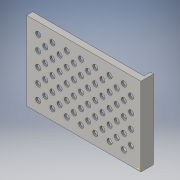
# Autodesk Inventor part: RaspPiCaseTop
Saved by Autodesk Inventor 2016 (Build 200138000, 138)
## iProperties
Created: 2016-04-29
Part Number: RaspPiCaseTop
Material: Generic
Document SubType Name: Modeling
Designer: mkepler
Density: 1 g/cm^3
Appearance: Default
Author: mkepler
Autodesk Inventor part; units mm, degrees
ref_plane "YZ Plane" through (0, 0, 0) normal (1, 0, 0) x (0, 1, 0)
ref_plane "XZ Plane" through (0, 0, 0) normal (0, 1, 0) x (-1, 0, 0)
ref_plane "XY Plane" through (0, 0, 0) normal (0, 0, 1) x (1, 0, 0)
sketch "Sketch1" plane through (0, 0, 0) normal (0, 1, 0) x (-1, 0, 0)
  line L0 (0, 0) -> (91.5, 0)
  line L1 (91.5, 0) -> (91.5, -63)
  line L2 (91.5, -63) -> (0, -63)
  circle A0 centre (84, -7.5) radius 2.15
  circle A1 centre (84, -19.5) radius 2.15
  circle A2 centre (84, -31.5) radius 2.15
  circle A3 centre (84, -55.5) radius 2.15
  circle A4 centre (84, -43.5) radius 2.15
  circle A5 centre (78, -13.5) radius 2.15
  circle A6 centre (78, -25.5) radius 2.15
  circle A7 centre (78, -37.5) radius 2.15
  circle A8 centre (78, -49.5) radius 2.15
  circle A9 centre (66, -13.5) radius 2.15
  circle A10 centre (66, -25.5) radius 2.15
  circle A11 centre (66, -37.5) radius 2.15
  circle A12 centre (66, -49.5) radius 2.15
  circle A13 centre (72, -31.5) radius 2.15
  circle A14 centre (72, -19.5) radius 2.15
  circle A15 centre (72, -7.5) radius 2.15
  circle A16 centre (72, -55.5) radius 2.15
  circle A17 centre (72, -43.5) radius 2.15
  line L3 (66, -55.5) -> (63, -55.5)
  line L4 (63, -55.5) -> (63, -45.305)
  circle A18 centre (42, -13.5) radius 2.15
  circle A19 centre (42, -25.5) radius 2.15
  circle A20 centre (42, -37.5) radius 2.15
  circle A21 centre (42, -49.5) radius 2.15
  circle A22 centre (48, -31.5) radius 2.15
  circle A23 centre (48, -19.5) radius 2.15
  circle A24 centre (48, -7.5) radius 2.15
  circle A25 centre (48, -55.5) radius 2.15
  circle A26 centre (48, -43.5) radius 2.15
  circle A27 centre (54, -37.5) radius 2.15
  circle A28 centre (60, -31.5) radius 2.15
  circle A29 centre (54, -25.5) radius 2.15
  circle A30 centre (60, -19.5) radius 2.15
  circle A31 centre (54, -13.5) radius 2.15
  circle A32 centre (60, -7.5) radius 2.15
  circle A33 centre (60, -43.5) radius 2.15
  circle A34 centre (54, -49.5) radius 2.15
  circle A35 centre (60, -55.5) radius 2.15
  line L5 (42, -55.5) -> (39, -55.5)
  line L6 (39, -55.5) -> (39, -51.65)
  circle A36 centre (6, -37.5) radius 2.15
  circle A37 centre (12, -31.5) radius 2.15
  circle A38 centre (6, -25.5) radius 2.15
  circle A39 centre (12, -19.5) radius 2.15
  circle A40 centre (6, -13.5) radius 2.15
  circle A41 centre (12, -7.5) radius 2.15
  circle A42 centre (12, -43.5) radius 2.15
  circle A43 centre (6, -49.5) radius 2.15
  circle A44 centre (12, -55.5) radius 2.15
  line L7 (12, -55.5) -> (15, -55.5)
  line L8 (15, -55.5) -> (15, -45.305)
  circle A45 centre (36, -43.5) radius 2.15
  circle A46 centre (30, -49.5) radius 2.15
  circle A47 centre (24, -55.5) radius 2.15
  circle A48 centre (24, -43.5) radius 2.15
  circle A49 centre (36, -55.5) radius 2.15
  circle A50 centre (36, -7.5) radius 2.15
  circle A51 centre (30, -25.5) radius 2.15
  circle A52 centre (30, -13.5) radius 2.15
  circle A53 centre (18, -25.5) radius 2.15
  circle A54 centre (24, -19.5) radius 2.15
  circle A55 centre (18, -13.5) radius 2.15
  circle A56 centre (24, -7.5) radius 2.15
  circle A57 centre (36, -19.5) radius 2.15
  circle A58 centre (36, -31.5) radius 2.15
  circle A59 centre (30, -37.5) radius 2.15
  circle A60 centre (24, -31.5) radius 2.15
  circle A61 centre (18, -49.5) radius 2.15
  circle A62 centre (18, -37.5) radius 2.15
  line L9 (36, -55.5) -> (39, -55.5)
  line L10 (0, 0) -> (0, -63)
  dimension "d0" = 91.5
  dimension "d1" = 63
  dimension "d2" = 4.3
  dimension "d3" = 7.5
  dimension "d4" = 7.5
  dimension "d11" = 4.3
  dimension "d17" = 3
  dimension "d18" = 3
  constraints: 63 centre point, 22 end point, 6 symmetric about line, 3 horizontal, 3 perpendicular, 1 parallel, 1 vertical
  measures "d0" distance of L1.end L2.end
  measures "d1" distance of L0.end L1.end
  measures "d2" diameter of A0
  measures "d3" distance from line of L0 A0.centre
  measures "d4" distance from line of L1 A0.centre
  measures "d11" diameter of A2
  measures "d17" distance of L3.start L3.end
  measures "d18" distance of L5.start L5.end
extrude "Extrusion1" add sketch "Sketch1" along normal blind 1.5
sketch "Sketch2" plane through (0, 1.5, 0) normal (0, 1, 0) x (1, 0, 0)
  line L0 (3, 0) -> (3, -3)
  line L1 (3, -3) -> (-94.5, -3)
  line L2 (-94.5, -3) -> (-94.5, 66)
  line L3 (-94.5, 66) -> (3, 66)
  line L4 (3, 66) -> (3, 0)
  line L5 (-91.5, 63) -> (-91.5, 0) projected
  line L6 (0, 63) -> (-91.5, 63) projected
  line L7 (-91.5, 0) -> (0, 0)
  line L8 (0, 0) -> (0, 63)
  line L9 (0, 63) -> (-91.5, 63)
  line L10 (-91.5, 63) -> (-91.5, 0)
  dimension "d30" = 97.5
  dimension "d31" = 69
  dimension "d32" = 97.5
  constraints: 18 end point, 3 perpendicular, 2 parallel, 1 horizontal, 1 vertical
  measures "d30" distance of L0.end L1.end
  measures "d31" distance of L1.end L2.end
  measures "d32" distance of L2.end L3.end
extrude "Extrusion2" add sketch "Sketch2" along normal blind 3.612 and the other way blind 1.5
sketch "Sketch5" plane through (0, 1.5, 0) normal (0, 1, 0) x (1, 0, 0)
  point P0 (0, 0)
sketch "Sketch6" plane through (0, 5.112, 0) normal (0, 1, 0) x (1, 0, 0)
  line L0 (0, 0) -> (0, 63) projected
  line L1 (3, 66) -> (3, -3) projected
  line L2 (0, 0) -> (3, 0)
  line L3 (3, 0) -> (3, 63)
  line L4 (3, 63) -> (0, 63)
  line L5 (0, 63) -> (0, 0)
  constraints: 8 end point, 2 parallel, 1 horizontal, 1 perpendicular, 1 point on line
extrude "Extrusion3" add sketch "Sketch6" along normal blind 5.388
sketch "Sketch7" plane through (-91.5, 1.5, -63) normal (0, 0, 1) x (1, 0, 0)
  point P0 (91.5, -1.5)
sketch "Sketch8" plane through (-91.5, 1.5, -63) normal (0, 0, 1) x (1, 0, 0)
  line L0 (91.5, 0) -> (0, 0) projected
  line L1 (0, 3.612) -> (91.5, 3.612) projected
  line L2 (0, 0) -> (91.5, 0)
  line L3 (91.5, 0) -> (91.5, 3.612)
  line L4 (91.5, 3.612) -> (0, 3.612)
  line L5 (0, 3.612) -> (0, 0)
  point P0 (91.5, -1.5)
  constraints: 8 end point, 2 parallel, 1 horizontal, 1 perpendicular
extrude "Extrusion4" cut sketch "Sketch8" against normal blind 0.5
sketch "Sketch9" plane through (0, 1.5, 0) normal (0, 0, -1) x (-1, 0, 0)
  line L0 (0, 3.612) -> (91.5, 3.612) projected
  line L1 (91.5, 0) -> (0, 0) projected
  line L2 (91.5, 3.612) -> (0, 3.612)
  line L3 (0, 3.612) -> (0, 0)
  line L4 (0, 0) -> (91.5, 0)
  line L5 (91.5, 0) -> (91.5, 3.612)
  point P0 (0, -1.5)
  constraints: 8 end point, 2 parallel, 1 horizontal, 1 perpendicular
extrude "Extrusion5" cut sketch "Sketch9" against normal blind 0.5
sketch "Sketch10" plane through (-91.5, 1.5, -63.5) normal (1, 0, 0) x (0, 0, -1)
  line L0 (0, 0) -> (0, 3.612) projected
  line L1 (0, 0) -> (-64, 0) projected
  line L2 (0, 3.612) -> (-64, 3.612)
  line L3 (-64, 3.612) -> (-64, 0)
  line L4 (-64, 0) -> (0, 0)
  line L5 (0, 0) -> (0, 3.612)
  point P0 (-63.5, -1.5)
  constraints: 8 end point, 2 parallel, 1 horizontal, 1 perpendicular
extrude "Extrusion6" cut sketch "Sketch10" against normal blind 0.5
sketch "Sketch11" plane through (3, 5.112, -63) normal (0, 0, -1) x (-1, 0, 0)
  line L0 (0, 5.388) -> (3, 5.388) projected
  line L1 (0, 0) -> (0, 5.388) projected
  line L2 (3, 5.388) -> (0, 5.388)
  line L3 (0, 5.388) -> (0, 0)
  line L4 (0, 0) -> (3, 0)
  line L5 (3, 0) -> (3, 5.388)
  point P0 (3, -5.112)
  constraints: 8 end point, 2 parallel, 1 horizontal, 1 perpendicular
extrude "Extrusion7" add sketch "Sketch11" along normal blind 3
sketch "Sketch12" plane through (0, 5.112, 0) normal (0, 0, 1) x (1, 0, 0)
  line L0 (0, 5.388) -> (3, 5.388) projected
  line L1 (-94.5, 0) -> (3, 0) projected
  line L2 (0, 5.388) -> (3, 5.388)
  line L3 (3, 5.388) -> (3, 0)
  line L4 (3, 0) -> (0, 0)
  line L5 (0, 0) -> (0, 5.388)
  point P0 (0, -5.112)
  constraints: 8 end point, 2 parallel, 1 horizontal, 1 perpendicular
extrude "Extrusion8" add sketch "Sketch12" along normal blind 3
sketch "Sketch13" plane through (0, 0, 0) normal (0, -1, 0) x (1, 0, 0)
  line L0 (-94.5, 3) -> (0, 3) projected
  line L1 (-94.5, 3) -> (-93.75, 3)
  line L2 (-93.75, 1.5) -> (2.25, 1.5)
  line L3 (2.25, 1.5) -> (2.25, -64.5)
  line L4 (2.25, -64.5) -> (-93.75, -64.5)
  line L5 (-93.75, -64.5) -> (-93.75, 1.5)
  line L6 (3, -66) -> (3, 3) projected
  line L7 (-94.5, 3) -> (3, 3)
  line L8 (3, 3) -> (3, -66)
  line L9 (3, -66) -> (-94.5, -66)
  line L10 (-94.5, -66) -> (-94.5, 3)
  point P0 (0, 0)
  dimension "d45" = 0.75
  dimension "d46" = 1.5
  dimension "d47" = 96
  dimension "d48" = 66
  constraints: 18 end point, 4 parallel, 2 horizontal, 2 perpendicular, 1 point on line
  measures "d45" distance of L0.start L1.end
  measures "d46" distance of L1.end L2.start
  measures "d47" distance of L3.end L4.end
  measures "d48" distance of L2.end L3.end
extrude "Extrusion9" cut sketch "Sketch13" against normal through all
sketch "Sketch14" plane through (-93.75, 0, -64.5) normal (-1, 0, 0) x (0, 0, 1)
  line L0 (0, 5.112) -> (66, 5.112) projected
  line L1 (0, 0) -> (0, 5.112) projected
  line L2 (66, 5.112) -> (0, 5.112)
  line L3 (0, 5.112) -> (0, 1.5)
  line L4 (0, 1.5) -> (66, 1.5)
  line L5 (66, 1.5) -> (66, 5.112)
  point P0 (64.5, 0)
  constraints: 8 end point, 2 parallel, 1 horizontal, 1 perpendicular, 1 point on line
extrude "Extrusion10" cut sketch "Sketch14" against normal through all
sketch "Sketch15" plane through (0, 10.5, 1.5) normal (0, 0, 1) x (1, 0, 0)
  line L0 (2.25, -5.388) -> (2.25, 0) projected
  line L1 (0, -5.388) -> (0, 0) projected
  line L2 (2.25, -5.388) -> (0, -5.388)
  line L3 (0, -5.388) -> (0, 0)
  line L4 (0, 0) -> (2.25, 0)
  line L5 (2.25, 0) -> (2.25, -5.388)
  point P0 (0, -10.5)
  constraints: 8 end point, 2 parallel, 1 horizontal, 1 perpendicular
extrude "Extrusion11" cut sketch "Sketch15" against normal through all
sketch "Sketch16" plane through (0, 1.5, 0) normal (0, 1, 0) x (1, 0, 0)
  line L0 (2.25, 64.5) -> (2.25, -1.5) projected
  line L1 (2.25, -1.5) -> (-0.75, -1.5)
  line L2 (-0.75, -1.5) -> (-0.75, 3.5)
  line L3 (-0.75, 3.5) -> (2.25, 3.5)
  line L4 (2.25, 3.5) -> (2.25, -1.5)
  line L5 (2.25, 64.5) -> (-0.75, 64.5)
  line L6 (-0.75, 64.5) -> (-0.75, 59.5)
  line L7 (-0.75, 59.5) -> (2.25, 59.5)
  line L8 (2.25, 59.5) -> (2.25, 64.5)
  line L9 (2.25, 3.5) -> (-0.75, 3.5)
  line L10 (-0.75, 3.5) -> (-0.75, 59.5)
  line L11 (-0.75, 59.5) -> (2.25, 59.5)
  line L12 (2.25, 59.5) -> (2.25, 3.5)
  point P0 (0, 0)
  dimension "d55" = 3
  dimension "d56" = 5
  dimension "d57" = 3
  dimension "d58" = 5
  constraints: 24 end point, 6 parallel, 3 horizontal, 3 perpendicular
  measures "d55" distance of L2.end L3.end
  measures "d56" distance of L1.end L2.end
  measures "d57" distance of L7.end L6.end
  measures "d58" distance of L6.end L5.end
extrude "Extrusion12" add sketch "Sketch16" along normal blind 9
sketch "Sketch17" plane through (0, 1.5, 0) normal (0, 1, 0) x (1, 0, 0)
  line L0 (-0.75, -1.5) -> (-93.75, -1.5) projected
  line L1 (-0.75, -1.5) -> (-0.75, 0)
  line L2 (-0.75, -1.5) -> (-0.75, 64.5) projected
  line L3 (-93.75, -1.5) -> (-93.75, 64.5) projected
  line L4 (-93.75, -1.5) -> (-93.75, 64.5)
  line L5 (-93.75, 64.5) -> (-0.75, 64.5) projected
  line L6 (-93.75, 64.5) -> (-0.75, 64.5)
  line L7 (-0.75, 64.5) -> (-0.75, 63)
  line L8 (-92.25, 63) -> (-0.75, 63)
  line L9 (-0.75, 0) -> (-92.25, 0)
  line L10 (-92.25, 0) -> (-92.25, 63)
  point P0 (0, 0)
  dimension "d61" = 1.5
  constraints: 14 end point, 3 perpendicular, 2 point on line, 1 collinear, 1 parallel
  measures "d61" distance of L2.end L7.end
extrude "Extrusion13" add sketch "Sketch17" along normal blind 3.65 contours L0 L3 L5 L2 L8 L10 L9 L1
sketch "Sketch18" plane through (-0.75, 1.5, 0) normal (0, 0, -1) x (-1, 0, 0)
  line L0 (91.5, 0) -> (91.5, 3.65) projected
  line L1 (0, 0) -> (0, 3.65) projected
  line L2 (91.5, 3.65) -> (0, 3.65)
  line L3 (0, 3.65) -> (0, 0)
  line L4 (0, 0) -> (91.5, 0)
  line L5 (91.5, 0) -> (91.5, 3.65)
  point P0 (-0.75, -1.5)
  constraints: 8 end point, 2 parallel, 1 horizontal, 1 perpendicular
extrude "Extrusion14" cut sketch "Sketch18" against normal blind 0.5
sketch "Sketch19" plane through (-92.25, 1.5, -63) normal (0, 0, 1) x (1, 0, 0)
  line L0 (91.5, 0) -> (0, 0) projected
  line L1 (0, 0) -> (0, 3.65) projected
  line L2 (91.5, 0) -> (0, 0)
  line L3 (0, 0) -> (0, 3.65)
  line L4 (0, 3.65) -> (91.5, 3.65)
  line L5 (91.5, 3.65) -> (91.5, 0)
  point P0 (92.25, -1.5)
  constraints: 8 end point, 2 parallel, 1 horizontal, 1 perpendicular
extrude "Extrusion15" cut sketch "Sketch19" against normal blind 0.5
sketch "Sketch20" plane through (-92.25, 1.5, 0.5) normal (1, 0, 0) x (0, 0, -1)
  line L0 (64, 0) -> (64, 3.65) projected
  line L1 (64, 0) -> (0, 0)
  line L2 (0, 0) -> (0, 3.65)
  line L3 (0, 3.65) -> (64, 3.65)
  line L4 (64, 3.65) -> (64, 0)
  point P0 (0.5, -1.5)
  constraints: 8 end point, 2 parallel, 1 horizontal, 1 perpendicular
extrude "Extrusion16" cut sketch "Sketch20" against normal blind 0.5
sketch "Sketch21" plane through (-0.75, 10.5, -64.5) normal (-1, 0, 0) x (0, 0, 1)
  line L0 (1, -5.35) -> (1, -9) projected
  line L1 (1, -9) -> (1, -5.35)
  line L2 (0, -5.35) -> (1, -5.35) projected
  line L3 (1, -5.35) -> (0, -5.35)
  line L4 (0, -5.35) -> (0, 0)
  line L5 (66, -5.35) -> (66, 0) projected
  line L6 (0, 0) -> (66, 0)
  line L7 (65, -5.35) -> (66, -5.35) projected
  line L8 (66, -5.4693) -> (65, -5.35)
  line L9 (65, -9) -> (65, -5.35) projected
  line L10 (65, -5.35) -> (65, -9)
  line L11 (65, -5.35) -> (66, -5.35)
  line L12 (66, -5.35) -> (66, 0)
  line L13 (65, -9) -> (1, -9) projected
  line L14 (65, -9) -> (1, -9)
  line L15 (1, -9) -> (1, -5.35)
  line L16 (1, -5.35) -> (0, -5.35)
  point P0 (64.5, -10.5)
  constraints: 22 end point, 4 perpendicular, 3 collinear, 2 horizontal, 1 vertical
extrude "Extrusion17" cut sketch "Sketch21" against normal blind 0.5
body "Solid1"
